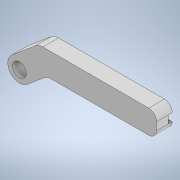
# Autodesk Inventor part: espcam-mount-2b
Saved by Autodesk Inventor 2020 (Build 240168000, 168)
## iProperties
Created: 2020-11-08
Part Number: espcam-mount-2b
Material: Generic
Document SubType Name: Modeling
Designer: alnwlsn
Density: 1 g/cm^3
Appearance: Default
Author: alnwlsn
Autodesk Inventor part; units mm, degrees
ref_plane "YZ Plane" through (0, 0, 0) normal (1, 0, 0) x (0, 1, 0)
ref_plane "XZ Plane" through (0, 0, 0) normal (0, 1, 0) x (-1, 0, 0)
ref_plane "XY Plane" through (0, 0, 0) normal (0, 0, 1) x (1, 0, 0)
sketch "Sketch1" plane through (0, 0, 0) normal (0, 0, 1) x (1, 0, 0)
  circle A0 centre (0, 0) radius 3
  line L0 (-1.9284, 2.2981) -> (4.0304, 7.2981)
  line L1 (5.9588, 8) -> (33, 8)
  line L2 (35, 6) -> (35, 4)
  line L3 (33, 2) -> (8.1426, 2)
  line L4 (6.2142, 1.2981) -> (1.9284, -2.2981)
  arc A1 (5.9588, 8) -> (4.0304, 7.2981) centre (5.9588, 5) ccw
  arc A2 (8.1426, 2) -> (6.2142, 1.2981) centre (8.1426, -1) ccw
  arc A3 (35, 6) -> (33, 8) centre (33, 6) ccw
  arc A4 (33, 2) -> (35, 4) centre (33, 4) ccw
  circle A5 centre (0, 0) radius 1.75
  point P0 (35, 8)
  point P1 (35, 2)
  dimension "d0" = 6
  dimension "d1" = 6
  dimension "d2" = 3
  dimension "d3" = 140
  dimension "d4" = 2
  dimension "d5" = 2
  dimension "d6" = 35
  dimension "d7" = 3.5
  constraints: 10 end point, 10 point on circle, 10 tangent, 6 centre point, 4 point on line, 2 coincident, 2 equal radius, 2 perpendicular, 1 horizontal, 1 parallel
  measures "d0" diameter of A0
  measures "d1" distance of point (35, 8) point (35, 2)
  measures "d2" radius of A1
  measures "d3" angle of L3 L4
  measures "d4" radius of A3
  measures "d5" distance from line of L3 point (0, 0)
  measures "d6" distance from line of point (0, 0) L2
  measures "d7" diameter of A5
extrude "Extrusion1" add sketch "Sketch1" along normal blind 4
sketch "Sketch3" plane through (0, 0, 0) normal (0, 0, -1) x (-1, 0, 0)
  line L0 (-63, 4) -> (-7, 4)
  line L1 (-7, 4) -> (-7, 6)
  line L2 (-7, 6) -> (-63, 6)
  line L3 (-63, 6) -> (-63, 4)
  line L4 (-35, 4) -> (-35, 6) projected
  line L5 (-63, 4) -> (-7, 6) construction
  line L6 (-7, 4) -> (-63, 6) construction
  point P0 (0, 0)
  point P1 (-35, 5)
  dimension "d14" = 28
  dimension "d15" = 2
  constraints: 12 end point, 3 midpoint, 2 parallel, 1 horizontal, 1 perpendicular
  measures "d14" distance from line of point (-35, 5) L1
  measures "d15" distance between parallel lines of L0 L2
extrude "Extrusion3" cut sketch "Sketch3" against normal blind 1
equation "\"d1\" = d0"
body "Solid1"
